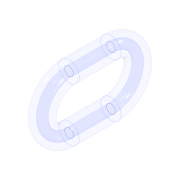
# Autodesk Inventor part: ring
Saved by Autodesk Inventor 2022 (Build 260153000, 153)
## iProperties
Created: 2022-06-02
Part Number: ring
Material: Generic
Document SubType Name: Modeling
Designer: Joseph Toombs
Density: 1 g/cm^3
Appearance: Default
Author: Joseph Toombs
Autodesk Inventor part; units mm, degrees
ref_plane "YZ Plane" through (0, 0, 0) normal (1, 0, 0) x (0, 1, 0)
ref_plane "XZ Plane" through (0, 0, 0) normal (0, 1, 0) x (-1, 0, 0)
ref_plane "XY Plane" through (0, 0, 0) normal (0, 0, 1) x (1, 0, 0)
sketch "Sketch1" plane through (0, 0, 0) normal (1, 0, 0) x (0, 1, 0)
  line L0 (0, -3.0812) -> (0, 3.0812) construction
  line L1 (3.939, -3.0812) -> (3.939, 3.0812)
  line L2 (-3.939, 3.0812) -> (-3.939, -3.0812)
  arc A0 (-3.939, -3.0812) -> (3.939, -3.0812) centre (0, -3.0812) ccw
  arc A1 (3.939, 3.0812) -> (-3.939, 3.0812) centre (0, 3.0812) ccw
  point P0 (0, 0)
  constraints: 8 end point, 4 point on circle, 4 tangent, 2 centre point, 1 midpoint, 1 parallel, 1 vertical
sketch "Sketch2" plane through (0, 0, 0) normal (0, 0, 1) x (1, 0, 0)
  circle A0 centre (0, 3.939) radius 1.5
  circle A1 centre (0, 3.939) radius 0.65
  circle A2 centre (0, 3.939) radius 0.64
  point P0 (0, 0)
  dimension "d0" = 3
  dimension "d1" = 1.3
  dimension "d2" = 0.01
  constraints: 3 centre point, 2 coincident
  measures "d0" diameter of A0
  measures "d1" diameter of A1
  measures "d2" radial gap between concentric circles of A1 A2
sweep "Sweep1" add profiles "Sketch2" path "Sketch1" contours A0
sweep "Sweep2" add profiles "Sketch2" path "Sketch1" separate body contours A2
sketch "Sketch3" plane through (0, 0, 0) normal (1, 0, 0) x (0, 1, 0)
  line L0 (7.1304, -9.2753) -> (0, -9.2753)
  line L1 (0, -9.2753) -> (0, -2.087)
  line L2 (0, -2.087) -> (7.1304, -2.087)
  line L3 (7.1304, -2.087) -> (7.1304, -9.2753)
  point P0 (0, 0)
  constraints: 8 end point, 2 parallel, 1 horizontal, 1 perpendicular
body "Solid1"
body "Solid2"
